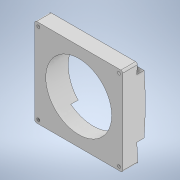
# Autodesk Inventor part: ventForDryer
Saved by Autodesk Inventor 2022.1 (Build 261234020, 234B)
## iProperties
Created: 2020-08-29
Part Number: ventForDryer
Material: Generic
Document SubType Name: Modeling
Designer: robst
Density: 1 g/cm^3
Appearance: Default
Author: robst
Autodesk Inventor part; units mm, degrees
ref_plane "YZ Plane" through (0, 0, 0) normal (1, 0, 0) x (0, 1, 0)
ref_plane "XZ Plane" through (0, 0, 0) normal (0, 1, 0) x (-1, 0, 0)
ref_plane "XY Plane" through (0, 0, 0) normal (0, 0, 1) x (1, 0, 0)
sketch "Sketch1" plane through (0, 0, 0) normal (1, 0, 0) x (0, 1, 0)
  line L0 (0, 0) -> (0, 12.7)
  line L1 (0, 0) -> (-101.6, 0) construction
  arc A0 (-101.6, 0) -> (0, 0) centre (-50.8, 607.4796) ccw
  line L2 (-50.8, -2.1204) -> (-50.8, 0) construction
  line L3 (0, 12.7) -> (101.6, 12.7) construction
  arc A1 (0, 12.7) -> (101.6, 12.7) centre (50.8, 620.1796) ccw
  line L4 (-101.6, 0) -> (-101.6, 12.7)
  line L5 (-101.6, 12.7) -> (-203.2, 12.7) construction
  arc A2 (-203.2, 12.7) -> (-101.6, 12.7) centre (-152.4, 620.1796) ccw
  line L6 (17.3591, 11.4976) -> (17.3591, 36.923)
  line L7 (17.3591, 36.923) -> (-135.0409, 36.923)
  line L8 (-135.0409, 36.923) -> (-135.0409, 10.8269)
  dimension "d0" = 12.7
  dimension "d1" = 101.6
  dimension "d3" = 50.8
  dimension "d4" = 2.1204
  dimension "d5" = 609.6
  dimension "d6" = 101.6
  dimension "d7" = 609.6
  dimension "d8" = 12.7
  dimension "d9" = 101.6
  dimension "d10" = 609.6
  dimension "d11" = 152.4
  dimension "d12" = 25.4254
  constraints: 18 end point, 9 point on circle, 4 horizontal, 3 centre point, 2 perpendicular, 2 vertical, 1 midpoint
  measures "d0" distance of L0.start L0.end
  measures "d1" distance of L0.start L1.end
  measures "d3" distance of L2.end L0.start
  measures "d4" distance of L2.start L2.end
  measures "d5" radius of A0
  measures "d6" distance of L0.end L3.end
  measures "d7" radius of A1
  measures "d8" distance of L1.end L4.end
  measures "d9" distance of L4.end L5.end
  measures "d10" radius of A2
  measures "d11" distance of L6.end L7.end
  measures "d12" distance of L6.start L6.end
extrude "Extrusion1" add sketch "Sketch1" along normal mid plane 152.4
sketch "Sketch3" plane through (-76.2, -135.0409, 36.923) normal (0, 0, 1) x (1, 0, 0)
  line L0 (0, 0) -> (0, 152.4) construction
  line L1 (152.4, 152.4) -> (152.4, 0) construction
  line L2 (0, 152.4) -> (152.4, 0) construction
  line L3 (152.4, 0) -> (0, 0) construction
  line L4 (152.4, 135.0409) -> (152.4, 152.4) construction
  line L5 (0, 0) -> (152.4, 152.4) construction
  circle A0 centre (76.2, 76.2) radius 57.15
  line L6 (6.35, 6.35) -> (146.05, 6.35) construction
  line L7 (146.05, 6.35) -> (146.05, 146.05) construction
  line L8 (146.05, 146.05) -> (6.35, 146.05) construction
  line L9 (6.35, 146.05) -> (6.35, 6.35) construction
  line L10 (6.35, 6.35) -> (146.05, 146.05) construction
  line L11 (146.05, 6.35) -> (6.35, 146.05) construction
  line L12 (0, 152.4) -> (152.4, 152.4) construction
  point P0 (76.2, 135.0409)
  dimension "d15" = 114.3
  dimension "d16" = 6.35
  dimension "d17" = 6.35
  constraints: 18 end point, 4 coincident, 3 midpoint, 3 perpendicular, 2 parallel, 1 centre point, 1 horizontal
  measures "d15" diameter of A0
  measures "d16" distance between parallel lines of L8 L12
  measures "d17" distance between parallel lines of L0 L9
extrude "Extrusion2" cut sketch "Sketch3" against normal through all
hole "Hole1" at (-69.85, 11.0091, 36.923) at (69.85, 11.0091, 36.923) at (69.85, -128.6909, 36.923) at (-69.85, -128.6909, 36.923) direction (0, 0, -1) diameter 5.1054 end through all clearance for "Hex Machine Screw" size "#10" standard "Ansi Unified Screw Threads"
fillet "Fillet1" radius 3.175 4 edges at (-76.2, 17.3591, 24.2103) (76.2, 17.3591, 24.2103) (76.2, -135.0409, 23.8749) (-76.2, -135.0409, 23.8749)
equation "\"d0\" = sidingDepth"
equation "\"d1\" = sidingHeight"
equation "\"d5\" = radiusOfCurvature"
equation "\"d6\" = sidingHeight"
equation "\"d7\" = radiusOfCurvature"
equation "\"d11\" = outsideWidthOfVent"
equation "\"d13\" = outsideWidthOfVent"
equation "\"d15\" = ventHole"
equation "\"sidingHeight\" = 101.6"
equation "\"sidingDepth\" = 12.7"
equation "\"radiusOfCurvature\" = 609.6"
equation "\"outsideWidthOfVent\" = 152.4"
equation "\"wallThicknessOfVent\" = 19.05"
equation "\"holeOffset\" = 6.35"
equation "\"ventHole\" = 114.3"
body "Solid1"
